Autodesk Fusion 360 part; units mm, degrees
(part 2 of 3)
  spline S36 degree 3 poles (-24.395426, -8.554265) (-24.395465, -8.554267) (-24.395536, -8.554312) (-24.395687, -8.554358) (-24.395947, -8.55446) (-24.39632, -8.554595) (-24.396767, -8.554761) (-24.397364, -8.55498) (-24.39811, -8.555255) (-24.399304, -8.555692) (-24.400799, -8.556237) (-24.402594, -8.556887) (-24.404391, -8.557534) (-24.406791, -8.558391) (-24.409796, -8.559455) (-24.413409, -8.560717) (-24.41824, -8.562383) (-24.4243, -8.56443) (-24.431601, -8.56683) (-24.438936, -8.569176) (-24.446305, -8.571466) (-24.456185, -8.574449) (-24.468619, -8.57804) (-24.483659, -8.582123) (-24.498834, -8.585986) (-24.519301, -8.590855) (-24.545236, -8.596386) (-24.576818, -8.602122) (-24.608947, -8.606975) (-24.641626, -8.610943) (-24.674857, -8.614028) (-24.708644, -8.616229) (-24.742988, -8.617551) (-24.780469, -8.617998) (-24.820659, -8.617471) (-24.876835, -8.6153) (-24.945324, -8.609872) (-25.025264, -8.598882) (-25.126818, -8.578556) (-25.247544, -8.542158) (-25.382434, -8.479922) (-25.505634, -8.399601) (-25.615962, -8.302262) (-25.71213, -8.190517) (-25.791503, -8.065677) (-25.85304, -7.928997) (-25.889046, -7.806726) (-25.914553, -7.676396) (-25.925922, -7.56615) (-25.929419, -7.42171) (-25.922149, -7.275178) (-25.893888, -7.104928) (-25.846241, -6.946475) (-25.779164, -6.799948) (-25.692713, -6.66553) (-25.623034, -6.584982) (-25.585516, -6.547045) knots 0 0 0 0 0.00001191 0.00002383 0.00004767 0.00009534 0.00014302 0.0001907 0.00028608 0.00038148 0.00057233 0.00076326 0.00095427 0.00114536 0.00152777 0.00191052 0.00229359 0.00306076 0.00382935 0.0045994 0.00537098 0.00614415 0.00769542 0.00925368 0.01081934 0.01239283 0.0155649 0.01877326 0.02202112 0.02531156 0.02864758 0.03203205 0.03546776 0.03895735 0.04327594 0.04752418 0.05582128 0.06387588 0.07171686 0.08687652 0.10158251 0.11613429 0.1308396 0.14557655 0.16021882 0.1750644 0.19040025 0.19833873 0.21488991 0.22356159 0.24167717 0.25880927 0.27521126 0.29116989 0.30699465 0.32300139 0.32300139 0.32300139 0.32300139
  spline S37 degree 3 poles (-25.585516, -6.547045) (-25.585469, -6.547019) (-25.585408, -6.546928) (-25.585253, -6.546786) (-25.584996, -6.54652) (-25.584621, -6.546149) (-25.584174, -6.5457) (-25.583577, -6.545104) (-25.582831, -6.544358) (-25.581635, -6.543167) (-25.580139, -6.541682) (-25.578341, -6.539903) (-25.57654, -6.53813) (-25.574135, -6.535772) (-25.571121, -6.532836) (-25.567491, -6.52933) (-25.562638, -6.524683) (-25.556542, -6.518921) (-25.549177, -6.512077) (-25.541764, -6.505308) (-25.534303, -6.498614) (-25.524299, -6.489793) (-25.511674, -6.478952) (-25.496325, -6.466233) (-25.480786, -6.453812) (-25.459829, -6.437659) (-25.433146, -6.418203) (-25.400347, -6.396037) (-25.366789, -6.375065) (-25.332474, -6.35529) (-25.297401, -6.336712) (-25.249516, -6.313481) (-25.187633, -6.287409) (-25.110548, -6.261018) (-25.03045, -6.239439) (-24.947346, -6.222675) (-24.83089, -6.206504) (-24.706133, -6.200325) (-24.576428, -6.204015) (-24.443025, -6.216082) (-24.315291, -6.240535) (-24.195161, -6.27832) (-24.110628, -6.312512) (-24.030429, -6.352955) (-23.954569, -6.399645) (-23.88306, -6.452573) (-23.815908, -6.511728) (-23.753121, -6.577091) (-23.714614, -6.624254) (-23.696116, -6.648755) knots 0 0 0 0 0.00001583 0.00003166 0.00006332 0.00012664 0.00018996 0.00025326 0.00037985 0.00050641 0.00075944 0.00101235 0.00126515 0.00151783 0.00202285 0.00252743 0.00303157 0.00403858 0.00504395 0.00604777 0.0070501 0.00805102 0.01004891 0.01204207 0.0140311 0.01601662 0.01997946 0.02393569 0.02789033 0.03184836 0.03581479 0.03979457 0.04781256 0.055942 0.06421981 0.07268094 0.08135818 0.09947342 0.11006808 0.12026679 0.1396396 0.14892549 0.15801382 0.16696446 0.17583997 0.18470439 0.1936219 0.20265543 0.21186547 0.21186547 0.21186547 0.21186547
  spline S38 degree 3 poles (-23.696116, -6.648755) (-23.696094, -6.648812) (-23.695999, -6.648897) (-23.695864, -6.649097) (-23.695601, -6.649434) (-23.69524, -6.649922) (-23.694801, -6.650505) (-23.694217, -6.651284) (-23.693488, -6.652258) (-23.692324, -6.653819) (-23.690871, -6.655773) (-23.689132, -6.658124) (-23.687398, -6.66048) (-23.685091, -6.66363) (-23.682219, -6.667582) (-23.678791, -6.672345) (-23.674243, -6.678729) (-23.668604, -6.686766) (-23.661915, -6.696493) (-23.655299, -6.70631) (-23.648756, -6.716216) (-23.640117, -6.729563) (-23.629502, -6.746475) (-23.617076, -6.767096) (-23.604944, -6.788075) (-23.593105, -6.809412) (-23.58156, -6.831107) (-23.566499, -6.860625) (-23.548409, -6.898443) (-23.527958, -6.945082) (-23.508681, -6.993157) (-23.490577, -7.042666) (-23.467785, -7.111241) (-23.442299, -7.200695) (-23.416694, -7.312775) (-23.395774, -7.430597) (-23.379532, -7.55417) (-23.365899, -7.706632) (-23.360337, -7.841833) (-23.359213, -7.984241) (-23.361184, -8.106853) (-23.370881, -8.296844) (-23.39479, -8.520005) (-23.444159, -8.769481) (-23.513751, -8.99517) (-23.603678, -9.196984) (-23.679006, -9.318219) (-23.719856, -9.373935) knots 0 0 0 0 0.00001823 0.00003647 0.00007294 0.0001459 0.00021888 0.00029186 0.00043785 0.00058389 0.0008761 0.00116849 0.00146105 0.00175379 0.00233982 0.00292658 0.0035141 0.00469142 0.00587191 0.00705566 0.00824278 0.00943337 0.01182537 0.0142325 0.01665555 0.01909531 0.02155255 0.02402802 0.02903642 0.03412638 0.03930334 0.04457246 0.04993864 0.06097948 0.07246123 0.08441435 0.0968659 0.10983987 0.13032478 0.1374365 0.15256362 0.16710419 0.19450011 0.2198151 0.24328444 0.26520232 0.28592841 0.28592841 0.28592841 0.28592841
  spline S39 degree 3 poles (-23.719856, -9.373935) (-23.71991, -9.373973) (-23.719966, -9.374101) (-23.720133, -9.374303) (-23.720323, -9.374573) (-23.720559, -9.37489) (-23.720871, -9.375315) (-23.721262, -9.375845) (-23.721888, -9.376693) (-23.722671, -9.377752) (-23.723612, -9.379021) (-23.724554, -9.380288) (-23.725811, -9.381975) (-23.727385, -9.38408) (-23.729279, -9.3866) (-23.731808, -9.389949) (-23.734981, -9.39412) (-23.738807, -9.399099) (-23.742651, -9.404053) (-23.746512, -9.40898) (-23.75168, -9.415509) (-23.758182, -9.423604) (-23.766061, -9.43322) (-23.774009, -9.44273) (-23.784684, -9.45525) (-23.798203, -9.47064) (-23.814727, -9.488709) (-23.831528, -9.506354) (-23.848606, -9.523575) (-23.865963, -9.540371) (-23.889436, -9.562165) (-23.91949, -9.58837) (-23.956721, -9.618165) (-23.995063, -9.64626) (-24.034514, -9.672655) (-24.088658, -9.705619) (-24.159327, -9.742656) (-24.248423, -9.780173) (-24.341926, -9.810837) (-24.439815, -9.834646) (-24.542078, -9.851609) (-24.648701, -9.861723) (-24.747073, -9.864653) (-24.834821, -9.862789) (-24.933295, -9.856099) (-25.05069, -9.839495) (-25.183656, -9.805449) (-25.306551, -9.757525) (-25.419202, -9.695724) (-25.487374, -9.64528) (-25.519396, -9.618055) knots 0 0 0 0 0.00001977 0.00003954 0.00007909 0.00011863 0.00015817 0.00023723 0.00031628 0.00047431 0.00063228 0.00079019 0.00094802 0.00126349 0.00157868 0.00189361 0.00252267 0.00315068 0.00377766 0.00440362 0.00502857 0.0062755 0.00751858 0.00875793 0.00999366 0.0124547 0.0149027 0.01733864 0.0197635 0.02217829 0.02458403 0.02937218 0.03413656 0.03888562 0.04362791 0.04837199 0.05789763 0.06753231 0.07734137 0.08738674 0.09772607 0.10841225 0.11949318 0.12723138 0.13473397 0.14909514 0.16273188 0.17582076 0.18856152 0.2011708 0.2011708 0.2011708 0.2011708
  spline S40 degree 3 poles (-25.519396, -9.618055) (-25.519451, -9.617994) (-25.519588, -9.617899) (-25.519834, -9.61768) (-25.520277, -9.617311) (-25.520903, -9.616775) (-25.521657, -9.616136) (-25.522659, -9.615281) (-25.52391, -9.614211) (-25.525906, -9.612496) (-25.528392, -9.610347) (-25.531362, -9.607758) (-25.534318, -9.60516) (-25.538238, -9.601684) (-25.543103, -9.597317) (-25.548887, -9.592035) (-25.556515, -9.58495) (-25.56591, -9.575999) (-25.576968, -9.565097) (-25.587798, -9.554045) (-25.5984, -9.542842) (-25.612215, -9.527724) (-25.628925, -9.508441) (-25.648089, -9.48467) (-25.666341, -9.460294) (-25.689459, -9.426989) (-25.716129, -9.383752) (-25.744449, -9.329455) (-25.769093, -9.272733) (-25.790057, -9.213591) (-25.80734, -9.152026) (-25.825721, -9.065562) (-25.833537, -8.998735) (-25.836416, -8.953505) knots 0 0 0 0 0.00002472 0.00004945 0.00009889 0.00019776 0.0002966 0.00039541 0.00059294 0.00079035 0.00118482 0.00157884 0.0019724 0.00236552 0.00315045 0.00393368 0.00471528 0.00627376 0.00782635 0.00937352 0.01091573 0.01245345 0.01551718 0.01856867 0.02161179 0.02465048 0.03072931 0.03683771 0.04300686 0.04926712 0.05564764 0.06217603 0.07577238 0.07577238 0.07577238 0.07577238
  line L18 (-25.836416, -8.953505) -> (-25.114226, -8.953505)
  spline S41 degree 3 poles (-25.114226, -8.953505) (-25.11419, -8.953651) (-25.114169, -8.953953) (-25.114074, -8.954546) (-25.113932, -8.955588) (-25.113713, -8.957071) (-25.113451, -8.958847) (-25.113093, -8.961207) (-25.112635, -8.964146) (-25.111878, -8.96882) (-25.110885, -8.974616) (-25.109616, -8.981513) (-25.108273, -8.988337) (-25.106389, -8.997303) (-25.103849, -9.00833) (-25.10049, -9.021325) (-25.095649, -9.038136) (-25.088861, -9.058451) (-25.079463, -9.081834) (-25.068871, -9.104039) (-25.057089, -9.125062) (-25.039898, -9.151358) (-25.015293, -9.18153) (-24.992387, -9.202475) (-24.980296, -9.212035) knots 0 0 0 0 0.00004513 0.00009023 0.00018037 0.00036035 0.00053995 0.00071917 0.00107647 0.00143227 0.00213939 0.00284064 0.00353611 0.00422592 0.00558893 0.00693059 0.00825183 0.01083675 0.01335229 0.01580753 0.01821221 0.0205767 0.02522625 0.02985048 0.02985048 0.02985048 0.02985048
  spline S42 degree 3 poles (-24.980296, -9.212035) (-24.98024, -9.212059) (-24.980157, -9.212156) (-24.979961, -9.212298) (-24.979632, -9.21257) (-24.979154, -9.212946) (-24.978582, -9.213401) (-24.977817, -9.214004) (-24.976858, -9.214756) (-24.975317, -9.215952) (-24.973379, -9.217436) (-24.971035, -9.219196) (-24.968672, -9.220937) (-24.965495, -9.223234) (-24.961476, -9.226058) (-24.956581, -9.229367) (-24.951611, -9.232598) (-24.946566, -9.235753) (-24.939725, -9.239866) (-24.93098, -9.244815) (-24.92021, -9.250433) (-24.909139, -9.255744) (-24.893881, -9.262459) (-24.874019, -9.270081) (-24.849141, -9.27794) (-24.823066, -9.284576) (-24.795795, -9.289992) (-24.767328, -9.294194) (-24.737664, -9.297183) (-24.712184, -9.298658) (-24.691216, -9.299244) (-24.673188, -9.299426) (-24.653232, -9.299089) (-24.624629, -9.297496) (-24.589832, -9.293544) (-24.549412, -9.285511) (-24.498098, -9.270573) (-24.437301, -9.243486) (-24.382506, -9.205403) (-24.337366, -9.16417) (-24.299649, -9.121493) (-24.274922, -9.08591) (-24.263196, -9.067085) knots 0 0 0 0 0.00001825 0.00003651 0.00007302 0.00014607 0.00021913 0.0002922 0.00043841 0.00058469 0.00087748 0.00117059 0.00146406 0.00175791 0.00234683 0.00293756 0.00353028 0.00412518 0.00472246 0.00592484 0.00713892 0.00836609 0.00960773 0.01213929 0.01474381 0.01743031 0.02020701 0.02308128 0.02605975 0.02914835 0.03073569 0.03235249 0.03455679 0.03672168 0.04094521 0.0450511 0.04906908 0.05696136 0.06489709 0.06896847 0.07528488 0.0819384 0.0819384 0.0819384 0.0819384
  spline S43 degree 3 poles (-24.263196, -9.067085) (-24.263147, -9.066977) (-24.263002, -9.066785) (-24.262763, -9.066376) (-24.262321, -9.06567) (-24.261702, -9.064654) (-24.260957, -9.063435) (-24.259967, -9.061803) (-24.258733, -9.059756) (-24.256768, -9.05646) (-24.254327, -9.05231) (-24.251431, -9.047284) (-24.248561, -9.042208) (-24.244762, -9.035354) (-24.240083, -9.026658) (-24.234592, -9.016047) (-24.229212, -9.005233) (-24.223942, -8.994216) (-24.217023, -8.979172) (-24.208654, -8.959849) (-24.199107, -8.935979) (-24.19, -8.911297) (-24.178306, -8.876904) (-24.164829, -8.831825) (-24.150594, -8.775109) (-24.138109, -8.715153) (-24.127368, -8.651956) (-24.118369, -8.585516) (-24.108476, -8.49056) (-24.104034, -8.417528) (-24.102136, -8.367785) knots 0 0 0 0 0.00003561 0.00007124 0.00014252 0.00028522 0.0004281 0.00057117 0.00085784 0.00114525 0.00172229 0.00230233 0.00288541 0.00347157 0.0046533 0.00584785 0.00705551 0.0082766 0.0095114 0.01202317 0.014593 0.01722287 0.01991463 0.02549015 0.03133236 0.03745197 0.04385828 0.05055936 0.05756225 0.07249603 0.07249603 0.07249603 0.07249603
  ellipse E2 centre (1150.427202, 948.865831) end of major axis (-13.478159, -21.350553) minor radius 28.956501 (-13.625826, -20.873205) -> (-13.473246, -21.356365) ccw
  spline S44 degree 3 poles (-13.473246, -21.356365) (-13.473203, -21.356392) (-13.473151, -21.356485) (-13.473011, -21.35663) (-13.472784, -21.356904) (-13.47245, -21.357284) (-13.472052, -21.357743) (-13.471521, -21.358354) (-13.470855, -21.359116) (-13.469789, -21.360332) (-13.468453, -21.361845) (-13.466843, -21.363653) (-13.465227, -21.365451) (-13.463065, -21.367834) (-13.460349, -21.37079) (-13.457063, -21.3743) (-13.452656, -21.378925) (-13.447086, -21.384612) (-13.4403, -21.391291) (-13.433419, -21.397818) (-13.426443, -21.404192) (-13.417028, -21.412475) (-13.405014, -21.422455) (-13.390196, -21.433835) (-13.374995, -21.444604) (-13.354214, -21.458147) (-13.32721, -21.473579) (-13.293279, -21.489621) (-13.257808, -21.503193) (-13.220801, -21.514291) (-13.182256, -21.522914) (-13.142173, -21.529062) (-13.100551, -21.532728) (-13.058754, -21.533904) (-13.017801, -21.532771) (-12.966494, -21.52815) (-12.90562, -21.516609) (-12.837479, -21.492778) (-12.775443, -21.459112) (-12.719626, -21.415643) (-12.687275, -21.380934) (-12.672226, -21.362295) knots 0 0 0 0 0.0000152 0.0000304 0.00006079 0.00012156 0.00018231 0.00024304 0.00036444 0.00048576 0.00072815 0.00097023 0.00121199 0.00145344 0.00193543 0.00241625 0.00289592 0.003852 0.004804 0.00575224 0.00669705 0.00763876 0.00951415 0.01138119 0.01324267 0.01510137 0.01882097 0.02256319 0.02635022 0.03020356 0.03414371 0.03818995 0.04236016 0.04667078 0.05072716 0.05464318 0.06211749 0.06924962 0.07621391 0.083197 0.09038387 0.09038387 0.09038387 0.09038387
  spline S45 degree 3 poles (-12.672226, -21.362295) (-12.672221, -21.362272) (-12.672176, -21.362241) (-12.672124, -21.362163) (-12.672015, -21.362035) (-12.671869, -21.361847) (-12.67169, -21.361624) (-12.671452, -21.361325) (-12.671155, -21.360952) (-12.67068, -21.360354) (-12.670088, -21.359605) (-12.669379, -21.358705) (-12.668672, -21.357802) (-12.667732, -21.356597) (-12.666562, -21.355085) (-12.665165, -21.353264) (-12.663312, -21.350826) (-12.661014, -21.34776) (-12.658287, -21.344052) (-12.65559, -21.340315) (-12.652922, -21.336549) (-12.649403, -21.331484) (-12.645078, -21.325078) (-12.640011, -21.317281) (-12.635064, -21.309366) (-12.628612, -21.298633) (-12.620844, -21.284916) (-12.612021, -21.268021) (-12.603675, -21.250656) (-12.595807, -21.232821) (-12.588417, -21.214516) (-12.579133, -21.189299) (-12.568738, -21.156541) (-12.558269, -21.115632) (-12.549712, -21.072837) (-12.543068, -21.028153) (-12.538331, -20.981578) (-12.535514, -20.933107) (-12.53459, -20.884412) (-12.535534, -20.836698) (-12.539453, -20.777064) (-12.549124, -20.706563) (-12.569038, -20.627415) (-12.592673, -20.566619) (-12.618371, -20.516533) (-12.644379, -20.475234) (-12.681753, -20.42818) (-12.728762, -20.382664) (-12.787141, -20.341886) (-12.852106, -20.310359) (-12.923533, -20.288054) (-13.001358, -20.274891) (-13.09578, -20.270209) (-13.176999, -20.276108) (-13.252832, -20.291712) (-13.310791, -20.309785) (-13.375015, -20.340819) (-13.432929, -20.380944) (-13.466838, -20.413326) (-13.482576, -20.430735) knots 0 0 0 0 0.00000715 0.00001431 0.00002862 0.00005725 0.00008587 0.0001145 0.00017176 0.00022903 0.00034359 0.00045817 0.00057278 0.00068743 0.0009168 0.0011463 0.00137593 0.0018356 0.00229584 0.00275669 0.00321819 0.00368038 0.00460695 0.00553671 0.00646995 0.00740696 0.00929337 0.01119826 0.0131238 0.01507212 0.01704527 0.01904521 0.02313256 0.0273489 0.03170726 0.03621948 0.04089625 0.04574722 0.05078106 0.05550411 0.06005954 0.06870514 0.0768121 0.08449091 0.08821165 0.09368971 0.09910183 0.10620576 0.11323827 0.12037497 0.12778318 0.13561204 0.14398747 0.15610626 0.15990029 0.16720338 0.17425492 0.18121652 0.18825692 0.18825692 0.18825692 0.18825692
  spline S46 degree 3 poles (-13.482576, -20.430735) (-13.482627, -20.430812) (-13.482768, -20.430938) (-13.483009, -20.43122) (-13.48345, -20.4317) (-13.484068, -20.432394) (-13.484812, -20.433226) (-13.4858, -20.434337) (-13.487031, -20.435731) (-13.48899, -20.43797) (-13.491419, -20.440786) (-13.494302, -20.444192) (-13.497154, -20.447625) (-13.500915, -20.452239) (-13.505538, -20.458075) (-13.51096, -20.465186) (-13.518027, -20.474819) (-13.52655, -20.487138) (-13.536267, -20.502341) (-13.545481, -20.517976) (-13.554194, -20.534045) (-13.565195, -20.556152) (-13.577695, -20.584933) (-13.59061, -20.621025) (-13.601521, -20.658844) (-13.613595, -20.712434) (-13.623467, -20.784087) (-13.625826, -20.842827) (-13.625826, -20.873205) knots 0 0 0 0 0.0000279 0.00005579 0.00011158 0.00022316 0.00033474 0.00044631 0.00066944 0.00089255 0.00133877 0.001785 0.00223128 0.00267766 0.00357082 0.00446482 0.00535996 0.0071548 0.00895787 0.01077156 0.01259824 0.01444021 0.0181784 0.02200385 0.02593251 0.02997909 0.03847552 0.04758904 0.04758904 0.04758904 0.04758904
  ellipse E3 centre (-5.783059, -31.50099) end of major axis (1.947224, -43.157824) minor radius 3.336725 (-13.346096, -19.759405) -> (-13.638536, -19.946735) ccw
  spline S47 degree 3 poles (-13.346096, -19.759405) (-13.345943, -19.759371) (-13.345658, -19.759234) (-13.345066, -19.759032) (-13.344334, -19.758756) (-13.343451, -19.758436) (-13.342274, -19.758006) (-13.340801, -19.757473) (-13.338442, -19.756623) (-13.335487, -19.75557) (-13.331933, -19.75432) (-13.328371, -19.753084) (-13.323606, -19.751453) (-13.317628, -19.749449) (-13.310423, -19.747101) (-13.300757, -19.74404) (-13.288584, -19.740351) (-13.27385, -19.736148) (-13.258974, -19.732165) (-13.243954, -19.7284) (-13.223675, -19.723657) (-13.197953, -19.718276) (-13.1666, -19.712708) (-13.134665, -19.708006) (-13.090973, -19.702849) (-13.046404, -19.699479) (-13.001045, -19.697797) (-12.963551, -19.697366) (-12.923291, -19.697885) (-12.866956, -19.700041) (-12.798256, -19.705425) (-12.718051, -19.716326) (-12.616146, -19.736485) (-12.495018, -19.772563) (-12.359664, -19.834267) (-12.236137, -19.913885) (-12.162529, -19.978213) (-12.128036, -20.012845) knots 0 0 0 0 0.00004693 0.00009387 0.00018776 0.00028168 0.00037561 0.00056355 0.00075159 0.00112793 0.00150464 0.00188174 0.00225922 0.00301539 0.0037732 0.00453272 0.00605709 0.00758897 0.00912881 0.01067706 0.01223416 0.01537652 0.01855933 0.02178578 0.02505896 0.03175648 0.03518688 0.03867491 0.04300442 0.04726431 0.05558625 0.06366654 0.0715326 0.08673495 0.10146408 0.11600988 0.13067364 0.13067364 0.13067364 0.13067364
  spline S48 degree 3 poles (-12.128036, -20.012845) (-12.128013, -20.012887) (-12.127928, -20.012944) (-12.127799, -20.013087) (-12.127555, -20.013323) (-12.127216, -20.013667) (-12.126805, -20.014077) (-12.126259, -20.014626) (-12.125577, -20.015312) (-12.124487, -20.01641) (-12.123128, -20.017784) (-12.1215, -20.019437) (-12.119877, -20.021092) (-12.11772, -20.023303) (-12.115033, -20.026073) (-12.111825, -20.02941) (-12.107573, -20.033873) (-12.1023, -20.039481) (-12.096038, -20.046259) (-12.089845, -20.053084) (-12.083721, -20.059954) (-12.07565, -20.069173) (-12.065731, -20.080812) (-12.054097, -20.094973) (-12.042735, -20.109319) (-12.027958, -20.128686) (-12.010161, -20.153373) (-11.989893, -20.183749) (-11.970721, -20.214867) (-11.952646, -20.246728) (-11.935667, -20.279332) (-11.914425, -20.32393) (-11.890596, -20.38166) (-11.866501, -20.453674) (-11.846806, -20.528648) (-11.831512, -20.60658) (-11.816751, -20.716092) (-11.811266, -20.830901) (-11.814237, -20.948177) (-11.82355, -21.065374) (-11.846795, -21.205355) (-11.894436, -21.363801) (-11.961513, -21.510332) (-12.047965, -21.64475) (-12.117646, -21.725298) (-12.155166, -21.763235) knots 0 0 0 0 0.00001451 0.00002903 0.00005806 0.00011611 0.00017416 0.0002322 0.00034827 0.00046431 0.00069633 0.00092825 0.00116008 0.00139182 0.00185502 0.00231787 0.00278037 0.00370437 0.0046271 0.00554863 0.00646902 0.00738836 0.00922414 0.01105658 0.01288626 0.01471378 0.01836458 0.02201391 0.02566655 0.02932729 0.03300088 0.036692 0.04414416 0.05172095 0.05945658 0.06738327 0.07553092 0.09259101 0.10178952 0.11071367 0.12784603 0.14424814 0.16020682 0.17603166 0.19203863 0.19203863 0.19203863 0.19203863
  spline S49 degree 3 poles (-12.155166, -21.763235) (-12.155212, -21.763261) (-12.155273, -21.763352) (-12.155428, -21.763494) (-12.155684, -21.76376) (-12.156057, -21.764131) (-12.156502, -21.76458) (-12.157097, -21.765176) (-12.157841, -21.765922) (-12.159032, -21.767113) (-12.160522, -21.768598) (-12.162314, -21.770377) (-12.164109, -21.77215) (-12.166505, -21.774508) (-12.169509, -21.777444) (-12.173125, -21.78095) (-12.177962, -21.785597) (-12.184037, -21.79136) (-12.191378, -21.798203) (-12.198768, -21.804972) (-12.206205, -21.811666) (-12.216179, -21.820487) (-12.228768, -21.831328) (-12.244076, -21.844048) (-12.259575, -21.856469) (-12.280482, -21.872621) (-12.307107, -21.892078) (-12.339842, -21.914245) (-12.373343, -21.935216) (-12.407607, -21.954991) (-12.442635, -21.973569) (-12.490471, -21.996802) (-12.552303, -22.022874) (-12.629343, -22.049264) (-12.70941, -22.070842) (-12.792492, -22.087607) (-12.87858, -22.099557) (-12.967668, -22.106701) (-13.063476, -22.109104) (-13.163638, -22.106265) (-13.297394, -22.094185) (-13.425517, -22.069697) (-13.546052, -22.031836) (-13.630903, -21.997554) (-13.71142, -21.956985) (-13.787592, -21.910128) (-13.859403, -21.856984) (-13.926839, -21.797559) (-13.989887, -21.731867) (-14.02854, -21.684452) (-14.047106, -21.659815) knots 0 0 0 0 0.0000158 0.0000316 0.00006321 0.00012641 0.0001896 0.00025279 0.00037915 0.00050547 0.00075804 0.00101049 0.00126282 0.00151504 0.00201915 0.00252282 0.00302605 0.00403127 0.00503488 0.00603695 0.00703756 0.00803678 0.01003136 0.0120213 0.01400722 0.01598974 0.01994687 0.02389784 0.02784764 0.03180128 0.03576374 0.03973997 0.04775209 0.05587719 0.06415198 0.07261123 0.08128746 0.09021082 0.099409 0.1100268 0.12025147 0.13968263 0.14900009 0.15812123 0.16710586 0.17601663 0.18491787 0.19387418 0.20294913 0.21220391 0.21220391 0.21220391 0.21220391
  spline S50 degree 3 poles (-14.047106, -21.659815) (-14.047128, -21.659758) (-14.047223, -21.659673) (-14.04736, -21.659473) (-14.047624, -21.659136) (-14.047988, -21.658648) (-14.048431, -21.658065) (-14.049018, -21.657286) (-14.049753, -21.656312) (-14.050926, -21.654752) (-14.05239, -21.652797) (-14.054142, -21.650447) (-14.05589, -21.64809) (-14.058214, -21.64494) (-14.061108, -21.640989) (-14.064561, -21.636226) (-14.067996, -21.631441) (-14.071412, -21.626634) (-14.075945, -21.62019) (-14.081565, -21.612079) (-14.088231, -21.602263) (-14.094823, -21.592357) (-14.103527, -21.579011) (-14.114222, -21.562101) (-14.126742, -21.541482) (-14.138966, -21.520505) (-14.150894, -21.499171) (-14.162527, -21.477479) (-14.177701, -21.447969) (-14.195926, -21.410164) (-14.216532, -21.36354) (-14.235955, -21.315487) (-14.254196, -21.266004) (-14.277156, -21.197483) (-14.302833, -21.108114) (-14.328633, -20.99616) (-14.349711, -20.878504) (-14.366076, -20.755146) (-14.379812, -20.603015) (-14.385419, -20.46814) (-14.38655, -20.3261) (-14.384576, -20.203794) (-14.37487, -20.014196) (-14.350914, -19.791389) (-14.3014, -19.542203) (-14.231519, -19.316654) (-14.141106, -19.11488) (-14.065326, -18.993714) (-14.024216, -18.938035) knots 0 0 0 0 0.00001828 0.00003657 0.00007314 0.0001463 0.00021947 0.00029265 0.00043904 0.00058547 0.00087847 0.00117163 0.00146497 0.00175848 0.00234603 0.0029343 0.0035233 0.00411304 0.00470355 0.00588688 0.0070734 0.00826321 0.00945642 0.01185344 0.01426527 0.01669273 0.01913659 0.02159763 0.02407659 0.02909102 0.03418575 0.03936621 0.04463752 0.05000459 0.06104314 0.07251706 0.0844566 0.09688856 0.10983668 0.13027045 0.13736168 0.15244997 0.16695826 0.19430734 0.2195969 0.24306072 0.26499326 0.28575655 0.28575655 0.28575655 0.28575655
  spline S51 degree 3 poles (-14.024216, -18.938035) (-14.024189, -18.938016) (-14.02416, -18.937951) (-14.024076, -18.93785) (-14.023942, -18.93766) (-14.023743, -18.937395) (-14.023508, -18.937074) (-14.023193, -18.936648) (-14.022799, -18.936115) (-14.022169, -18.935263) (-14.02138, -18.934198) (-14.020433, -18.932923) (-14.019484, -18.931649) (-14.018218, -18.929953) (-14.016633, -18.927837) (-14.014727, -18.925305) (-14.01218, -18.921938) (-14.008985, -18.917746) (-14.005133, -18.912741) (-14.001263, -18.907763) (-13.997376, -18.902811) (-13.992175, -18.89625) (-13.985631, -18.888114) (-13.977702, -18.878451) (-13.969704, -18.868895) (-13.958963, -18.856315) (-13.945364, -18.840853) (-13.928745, -18.822701) (-13.91185, -18.804977) (-13.89468, -18.78768) (-13.877233, -18.770812) (-13.853642, -18.748929) (-13.823445, -18.72262) (-13.786043, -18.692712) (-13.747534, -18.664516) (-13.707919, -18.638034) (-13.653563, -18.604968) (-13.582629, -18.567829) (-13.493211, -18.530222) (-13.39938, -18.499499) (-13.301151, -18.475655) (-13.198532, -18.458675) (-13.091528, -18.448557) (-12.993035, -18.445631) (-12.905433, -18.447479) (-12.807516, -18.454103) (-12.690802, -18.470551) (-12.558603, -18.504315) (-12.436406, -18.551889) (-12.324357, -18.613299) (-12.256535, -18.66345) (-12.224666, -18.690525) knots 0 0 0 0 0.00000994 0.00001988 0.00003978 0.00007955 0.00011933 0.0001591 0.00023862 0.00031813 0.00047709 0.00063598 0.00079481 0.00095356 0.00127086 0.00158788 0.00190463 0.0025373 0.0031689 0.00379944 0.00442893 0.00505739 0.00631127 0.00756118 0.00880726 0.01004961 0.01252362 0.01498419 0.01743233 0.01986904 0.02229533 0.02471223 0.02952182 0.0343065 0.03907489 0.04383565 0.04859751 0.05815709 0.06782455 0.07766628 0.08774516 0.09811974 0.10884363 0.11996535 0.1276613 0.13512168 0.1493991 0.16295401 0.17596474 0.18863321 0.20117846 0.20117846 0.20117846 0.20117846
  spline S52 degree 3 poles (-12.224666, -18.690525) (-12.224611, -18.690586) (-12.224474, -18.69068) (-12.224229, -18.690898) (-12.223788, -18.691265) (-12.223165, -18.691798) (-12.222415, -18.692435) (-12.221417, -18.693285) (-12.220172, -18.694349) (-12.218185, -18.696056) (-12.21571, -18.698194) (-12.212754, -18.700771) (-12.209812, -18.703357) (-12.205911, -18.706817) (-12.20107, -18.711166) (-12.195315, -18.716426) (-12.187725, -18.723483) (-12.17838, -18.732403) (-12.167384, -18.743272) (-12.156617, -18.754295) (-12.146079, -18.765472) (-12.132349, -18.780564) (-12.115747, -18.799825) (-12.096715, -18.823582) (-12.078596, -18.847959) (-12.055646, -18.881297) (-12.029181, -18.924615) (-12.001093, -18.979048) (-11.976646, -19.035956) (-11.955833, -19.095332) (-11.93864, -19.157178) (-11.920279, -19.244108) (-11.91236, -19.311288) (-11.909346, -19.356775) knots 0 0 0 0 0.0000246 0.00004921 0.00009842 0.00019682 0.00029519 0.00039353 0.00059012 0.00078659 0.0011792 0.00157136 0.00196308 0.00235436 0.00313564 0.00391527 0.0046933 0.00624481 0.00779065 0.00933132 0.0108673 0.01239908 0.01545192 0.01849396 0.02152923 0.02456179 0.03063395 0.0367436 0.04292214 0.04919979 0.05560524 0.06216532 0.07584137 0.07584137 0.07584137 0.07584137
  line L19 (-11.909346, -19.356775) -> (-12.626456, -19.354225)
  spline S53 degree 3 poles (-12.626456, -19.354225) (-12.626492, -19.35408) (-12.626516, -19.35378) (-12.626614, -19.353191) (-12.626764, -19.352158) (-12.626994, -19.350686) (-12.627269, -19.348923) (-12.627642, -19.346581) (-12.62812, -19.343666) (-12.628907, -19.339031) (-12.629935, -19.333284) (-12.631242, -19.326447) (-12.63262, -19.319685) (-12.634544, -19.310807) (-12.637125, -19.299894) (-12.640521, -19.287041) (-12.645394, -19.270433) (-12.652192, -19.250387) (-12.661574, -19.227343) (-12.672122, -19.205496) (-12.683844, -19.184848) (-12.700945, -19.159068) (-12.725462, -19.129551) (-12.74831, -19.109195) (-12.760376, -19.099935) knots 0 0 0 0 0.00004484 0.00008967 0.00017923 0.00035807 0.00053651 0.00071456 0.00106948 0.00142284 0.00212493 0.00282093 0.00351095 0.00419508 0.00554613 0.006875 0.00818265 0.01073811 0.01322147 0.01564229 0.01801099 0.02033878 0.02491669 0.0294796 0.0294796 0.0294796 0.0294796
  spline S54 degree 3 poles (-12.760376, -19.099935) (-12.760431, -19.099913) (-12.760514, -19.099819) (-12.76071, -19.099684) (-12.761039, -19.099423) (-12.761518, -19.099064) (-12.762089, -19.098629) (-12.762855, -19.098051) (-12.763814, -19.097332) (-12.765356, -19.096188) (-12.767296, -19.094768) (-12.769642, -19.093084) (-12.772007, -19.091417) (-12.775189, -19.089218) (-12.779216, -19.086514) (-12.784121, -19.083345) (-12.79078, -19.079207) (-12.799302, -19.074215) (-12.809812, -19.068532) (-12.820631, -19.063141) (-12.831759, -19.058042) (-12.847119, -19.051585) (-12.867128, -19.044252) (-12.892198, -19.036687) (-12.918501, -19.03029) (-12.946034, -19.025063) (-12.9748, -19.021002) (-13.004797, -19.01811) (-13.030575, -19.016681) (-13.051802, -19.016113) (-13.069997, -19.015934) (-13.09008, -19.016273) (-13.118778, -19.017882) (-13.153651, -19.02187) (-13.194108, -19.029972) (-13.245345, -19.045014) (-13.30589, -19.072256) (-13.360256, -19.110536) (-13.404826, -19.151912) (-13.441898, -19.194675) (-13.466064, -19.230295) (-13.477486, -19.249125) knots 0 0 0 0 0.00001795 0.0000359 0.0000718 0.00014363 0.00021549 0.00028737 0.00043122 0.00057519 0.00086348 0.00115226 0.00144157 0.00173142 0.00231282 0.00289668 0.00348316 0.00466468 0.00585883 0.00706699 0.00829044 0.00953048 0.0120648 0.01467936 0.01738248 0.02018166 0.02308367 0.02609459 0.02921985 0.03082698 0.03246447 0.03467839 0.03685122 0.0410857 0.04519638 0.04921342 0.05708839 0.06498957 0.06903834 0.07531483 0.08192171 0.08192171 0.08192171 0.08192171
  spline S55 degree 3 poles (-13.477486, -19.249125) (-13.477534, -19.249233) (-13.477675, -19.249427) (-13.477911, -19.249838) (-13.478345, -19.250547) (-13.478952, -19.251569) (-13.479684, -19.252794) (-13.480657, -19.254435) (-13.481869, -19.256493) (-13.483801, -19.259804) (-13.486199, -19.263975) (-13.489047, -19.269022) (-13.491868, -19.27412) (-13.495604, -19.281001) (-13.500208, -19.289729) (-13.505612, -19.300373) (-13.512716, -19.31491) (-13.521327, -19.333589) (-13.531181, -19.356676) (-13.540613, -19.38056) (-13.549623, -19.405239) (-13.561208, -19.439607) (-13.574595, -19.484614) (-13.588796, -19.541195) (-13.601318, -19.600965) (-13.612166, -19.663927) (-13.621343, -19.730085) (-13.631572, -19.824578) (-13.636367, -19.897244) (-13.638536, -19.946735) knots 0 0 0 0 0.00003558 0.00007117 0.00014239 0.00028496 0.00042771 0.00057065 0.00085707 0.00114422 0.00172076 0.00230031 0.00288291 0.00346859 0.00464936 0.00584293 0.00704959 0.00950322 0.01201248 0.01457938 0.01720578 0.01989345 0.02545867 0.03128727 0.03738958 0.04377463 0.05045029 0.05742351 0.07228503 0.07228503 0.07228503 0.07228503
  line L20 (-30.972226, -31.397235) -> (-31.109706, -31.317855)
  spline S56 degree 3 poles (-31.109706, -31.317855) (-31.109736, -31.317824) (-31.109821, -31.317794) (-31.109965, -31.317701) (-31.11023, -31.317553) (-31.1106, -31.317333) (-31.111046, -31.317071) (-31.111637, -31.316717) (-31.112372, -31.316272) (-31.113539, -31.315551) (-31.114983, -31.314633) (-31.116693, -31.313506) (-31.118377, -31.312353) (-31.120587, -31.310785) (-31.123287, -31.308765) (-31.12643, -31.306243) (-31.130475, -31.302766) (-31.13528, -31.298199) (-31.140639, -31.292379) (-31.145571, -31.286258) (-31.150071, -31.27986) (-31.155476, -31.27101) (-31.161133, -31.259361) (-31.166086, -31.244664) (-31.169146, -31.229456) (-31.170635, -31.208723) (-31.167406, -31.182263) (-31.159234, -31.162399) (-31.153856, -31.153085) knots 0 0 0 0 0.00001296 0.00002591 0.00005181 0.00010357 0.00015528 0.00020695 0.00031013 0.00041314 0.0006186 0.00082337 0.00102747 0.00123094 0.00163605 0.00203893 0.00243978 0.00323597 0.0040261 0.00481132 0.00559265 0.00637096 0.00792065 0.00946615 0.01101166 0.01256136 0.01568806 0.01891458 0.01891458 0.01891458 0.01891458
  line L21 (-31.153856, -31.153085) -> (-30.024486, -29.196945)
  spline S57 degree 3 poles (-30.024486, -29.196945) (-30.024455, -29.196915) (-30.024425, -29.19683) (-30.024332, -29.196685) (-30.024184, -29.196421) (-30.023964, -29.196051) (-30.023701, -29.195605) (-30.023348, -29.195014) (-30.022902, -29.194279) (-30.022181, -29.193112) (-30.021263, -29.191668) (-30.020135, -29.189958) (-30.018982, -29.188273) (-30.017414, -29.186064) (-30.015393, -29.183364) (-30.01287, -29.180221) (-30.009393, -29.176175) (-30.004825, -29.17137) (-29.999005, -29.166012) (-29.992883, -29.161079) (-29.986484, -29.156579) (-29.977633, -29.151174) (-29.965983, -29.145518) (-29.951286, -29.140565) (-29.936078, -29.137505) (-29.915344, -29.136015) (-29.888884, -29.139244) (-29.869019, -29.147417) (-29.859706, -29.152795) knots 0 0 0 0 0.00001296 0.00002591 0.00005181 0.00010358 0.00015529 0.00020696 0.00031016 0.00041317 0.00061865 0.00082343 0.00102755 0.00123104 0.00163618 0.00203909 0.00243997 0.00323623 0.00402641 0.00481169 0.00559308 0.00637144 0.00792121 0.00946679 0.01101235 0.01256208 0.01568881 0.01891534 0.01891534 0.01891534 0.01891534
  line L22 (-29.859706, -29.152795) -> (-29.722226, -29.232165)
  spline S58 degree 3 poles (-29.722226, -29.232165) (-29.722195, -29.232196) (-29.72211, -29.232226) (-29.721966, -29.232319) (-29.721702, -29.232467) (-29.721331, -29.232687) (-29.720886, -29.23295) (-29.720295, -29.233303) (-29.71956, -29.233748) (-29.718392, -29.23447) (-29.716948, -29.235388) (-29.715239, -29.236516) (-29.713554, -29.237669) (-29.711345, -29.239237) (-29.708645, -29.241257) (-29.705501, -29.24378) (-29.701456, -29.247257) (-29.696651, -29.251825) (-29.691293, -29.257646) (-29.68636, -29.263768) (-29.68186, -29.270166) (-29.676455, -29.279017) (-29.670798, -29.290667) (-29.665845, -29.305365) (-29.662786, -29.320573) (-29.661296, -29.341307) (-29.664525, -29.367767) (-29.672697, -29.387631) (-29.678076, -29.396945) knots 0 0 0 0 0.00001296 0.00002591 0.00005181 0.00010358 0.00015529 0.00020696 0.00031016 0.00041317 0.00061865 0.00082343 0.00102755 0.00123104 0.00163618 0.00203909 0.00243997 0.00323623 0.00402641 0.00481169 0.00559308 0.00637144 0.00792121 0.00946679 0.01101235 0.01256208 0.01568881 0.01891534 0.01891534 0.01891534 0.01891534
  line L23 (-29.678076, -29.396945) -> (-30.807446, -31.353085)
  spline S59 degree 3 poles (-30.807446, -31.353085) (-30.807476, -31.353115) (-30.807506, -31.3532) (-30.807599, -31.353345) (-30.807747, -31.353609) (-30.807968, -31.353979) (-30.80823, -31.354425) (-30.808584, -31.355016) (-30.809029, -31.355751) (-30.809751, -31.356918) (-30.810668, -31.358362) (-30.811796, -31.360072) (-30.812949, -31.361757) (-30.814517, -31.363966) (-30.816538, -31.366666) (-30.819061, -31.369809) (-30.822538, -31.373854) (-30.827106, -31.378659) (-30.832926, -31.384017) (-30.839048, -31.388949) (-30.845447, -31.393449) (-30.854298, -31.398853) (-30.865948, -31.404509) (-30.880646, -31.409461) (-30.895854, -31.412521) (-30.916587, -31.41401) (-30.943047, -31.410782) (-30.962912, -31.402612) (-30.972226, -31.397235) knots 0 0 0 0 0.00001296 0.00002591 0.00005181 0.00010358 0.00015529 0.00020696 0.00031016 0.00041317 0.00061865 0.00082343 0.00102755 0.00123103 0.00163617 0.00203907 0.00243994 0.00323617 0.00402634 0.00481159 0.00559296 0.0063713 0.00792103 0.00946659 0.01101214 0.01256187 0.01568859 0.01891498 0.01891498 0.01891498 0.01891498
  line L24 (-19.427876, -11.401835) -> (-19.565356, -11.322455)
  spline S60 degree 3 poles (-19.565356, -11.322455) (-19.565386, -11.322424) (-19.565471, -11.322394) (-19.565615, -11.322301) (-19.56588, -11.322153) (-19.56625, -11.321933) (-19.566696, -11.321671) (-19.567287, -11.321317) (-19.568022, -11.320872) (-19.569189, -11.320151) (-19.570633, -11.319233) (-19.572343, -11.318106) (-19.574027, -11.316953) (-19.576237, -11.315385) (-19.578937, -11.313365) (-19.58208, -11.310843) (-19.586125, -11.307366) (-19.59093, -11.302799) (-19.596289, -11.296979) (-19.601221, -11.290858) (-19.605721, -11.28446) (-19.611126, -11.27561) (-19.616783, -11.263961) (-19.621736, -11.249264) (-19.624796, -11.234056) (-19.626285, -11.213323) (-19.623056, -11.186863) (-19.614884, -11.166999) (-19.609506, -11.157685) knots 0 0 0 0 0.00001296 0.00002591 0.00005181 0.00010357 0.00015528 0.00020695 0.00031013 0.00041314 0.0006186 0.00082337 0.00102747 0.00123094 0.00163605 0.00203893 0.00243978 0.00323597 0.0040261 0.00481132 0.00559265 0.00637096 0.00792065 0.00946615 0.01101166 0.01256136 0.01568806 0.01891458 0.01891458 0.01891458 0.01891458
  line L25 (-19.609506, -11.157685) -> (-18.480136, -9.201545)
  spline S61 degree 3 poles (-18.480136, -9.201545) (-18.480105, -9.201515) (-18.480075, -9.20143) (-18.479982, -9.201285) (-18.479834, -9.201021) (-18.479614, -9.200651) (-18.479351, -9.200205) (-18.478998, -9.199614) (-18.478552, -9.198879) (-18.477831, -9.197712) (-18.476913, -9.196268) (-18.475785, -9.194558) (-18.474632, -9.192873) (-18.473064, -9.190664) (-18.471043, -9.187964) (-18.46852, -9.184821) (-18.465043, -9.180775) (-18.460475, -9.17597) (-18.454655, -9.170612) (-18.448533, -9.165679) (-18.442134, -9.161179) (-18.433283, -9.155774) (-18.421633, -9.150118) (-18.406936, -9.145165) (-18.391728, -9.142105) (-18.370994, -9.140615) (-18.344534, -9.143844) (-18.324669, -9.152017) (-18.315356, -9.157395) knots 0 0 0 0 0.00001296 0.00002591 0.00005181 0.00010358 0.00015529 0.00020696 0.00031016 0.00041317 0.00061865 0.00082343 0.00102755 0.00123104 0.00163618 0.00203909 0.00243997 0.00323623 0.00402641 0.00481169 0.00559308 0.00637144 0.00792121 0.00946679 0.01101235 0.01256208 0.01568881 0.01891534 0.01891534 0.01891534 0.01891534
  line L26 (-18.315356, -9.157395) -> (-18.177876, -9.236765)
  spline S62 degree 3 poles (-18.177876, -9.236765) (-18.177845, -9.236796) (-18.17776, -9.236826) (-18.177616, -9.236919) (-18.177352, -9.237067) (-18.176981, -9.237287) (-18.176536, -9.23755) (-18.175945, -9.237903) (-18.17521, -9.238348) (-18.174042, -9.23907) (-18.172598, -9.239988) (-18.170889, -9.241116) (-18.169204, -9.242269) (-18.166995, -9.243837) (-18.164295, -9.245857) (-18.161151, -9.24838) (-18.157106, -9.251857) (-18.152301, -9.256425) (-18.146943, -9.262246) (-18.14201, -9.268368) (-18.13751, -9.274766) (-18.132105, -9.283617) (-18.126448, -9.295267) (-18.121495, -9.309965) (-18.118436, -9.325173) (-18.116946, -9.345907) (-18.120175, -9.372367) (-18.128347, -9.392231) (-18.133726, -9.401545) knots 0 0 0 0 0.00001296 0.00002591 0.00005181 0.00010358 0.00015529 0.00020696 0.00031016 0.00041317 0.00061865 0.00082343 0.00102755 0.00123104 0.00163618 0.00203909 0.00243997 0.00323623 0.00402641 0.00481169 0.00559308 0.00637144 0.00792121 0.00946679 0.01101235 0.01256208 0.01568881 0.01891534 0.01891534 0.01891534 0.01891534
  line L27 (-18.133726, -9.401545) -> (-19.263096, -11.357685)
  spline S63 degree 3 poles (-19.263096, -11.357685) (-19.263126, -11.357715) (-19.263156, -11.3578) (-19.263249, -11.357945) (-19.263397, -11.358209) (-19.263618, -11.358579) (-19.26388, -11.359025) (-19.264234, -11.359616) (-19.264679, -11.360351) (-19.265401, -11.361518) (-19.266318, -11.362962) (-19.267446, -11.364672) (-19.268599, -11.366357) (-19.270167, -11.368566) (-19.272188, -11.371266) (-19.274711, -11.374409) (-19.278188, -11.378454) (-19.282756, -11.383259) (-19.288576, -11.388617) (-19.294698, -11.393549) (-19.301097, -11.398049) (-19.309948, -11.403453) (-19.321598, -11.409109) (-19.336296, -11.414061) (-19.351504, -11.417121) (-19.372237, -11.41861) (-19.398697, -11.415382) (-19.418562, -11.407212) (-19.427876, -11.401835) knots 0 0 0 0 0.00001296 0.00002591 0.00005181 0.00010358 0.00015529 0.00020696 0.00031016 0.00041317 0.00061865 0.00082343 0.00102755 0.00123103 0.00163617 0.00203907 0.00243994 0.00323617 0.00402634 0.00481159 0.00559296 0.0063713 0.00792103 0.00946659 0.01101214 0.01256187 0.01568859 0.01891498 0.01891498 0.01891498 0.01891498
  line L28 (-35.684336, -26.743225) -> (-35.763716, -26.605745)
  spline S64 degree 3 poles (-35.763716, -26.605745) (-35.763711, -26.605742) (-35.763739, -26.60572) (-35.763746, -26.605685) (-35.763794, -26.605613) (-35.763844, -26.605521) (-35.76391, -26.605408) (-35.763995, -26.605258) (-35.764102, -26.605071) (-35.764272, -26.604771) (-35.764484, -26.604396) (-35.764735, -26.603944) (-35.764985, -26.603492) (-35.765314, -26.602889) (-35.765721, -26.602134) (-35.7662, -26.601224) (-35.766828, -26.600009) (-35.767591, -26.598484) (-35.768473, -26.596644) (-35.769322, -26.594794) (-35.770136, -26.592936) (-35.771176, -26.590451) (-35.772391, -26.587325) (-35.773718, -26.583541) (-35.774912, -26.579732) (-35.776324, -26.574635) (-35.777764, -26.568214) (-35.778974, -26.560446) (-35.779672, -26.552656) (-35.779864, -26.544867) (-35.779556, -26.537105) (-35.778491, -26.526834) (-35.775942, -26.514165) (-35.770989, -26.499467) (-35.764197, -26.485473) (-35.755608, -26.472381) (-35.741751, -26.456282) (-35.72888, -26.446343) (-35.719566, -26.440965) knots 0 0 0 0 0.00000162 0.00000648 0.00001296 0.00002591 0.00003886 0.00005181 0.00007769 0.00010357 0.00015528 0.00020695 0.00025856 0.00031013 0.00041314 0.00051596 0.0006186 0.00082338 0.00102748 0.00123095 0.00143381 0.00163608 0.00203896 0.00243981 0.00283881 0.00323614 0.00402628 0.00481152 0.00559287 0.00637121 0.00714727 0.00792172 0.00946727 0.01101283 0.01256256 0.01412145 0.01569602 0.01892257 0.01892257 0.01892257 0.01892257
  line L29 (-35.719566, -26.440965) -> (-33.763426, -25.311595)
  spline S65 degree 3 poles (-33.763426, -25.311595) (-33.763384, -25.311584) (-33.763315, -25.311525) (-33.763163, -25.311447) (-33.762902, -25.311292) (-33.762527, -25.311081) (-33.762076, -25.310827) (-33.761475, -25.310491) (-33.760721, -25.310077) (-33.759513, -25.309427) (-33.757996, -25.308635) (-33.756165, -25.307718) (-33.754324, -25.306836) (-33.751862, -25.305706) (-33.748762, -25.304378) (-33.745006, -25.302917) (-33.739972, -25.301151) (-33.733614, -25.299274) (-33.725895, -25.297543) (-33.718127, -25.296332) (-33.710336, -25.295634) (-33.699969, -25.295379) (-33.687051, -25.296305) (-33.671847, -25.299364) (-33.657146, -25.304319) (-33.638445, -25.313396) (-33.617143, -25.329422) (-33.604024, -25.346431) (-33.598646, -25.355745) knots 0 0 0 0 0.00001296 0.00002591 0.00005181 0.00010358 0.00015529 0.00020696 0.00031016 0.00041317 0.00061864 0.00082343 0.00102754 0.00123102 0.00163616 0.00203906 0.00243992 0.00323615 0.0040263 0.00481154 0.0055929 0.00637123 0.00792096 0.00946652 0.0110121 0.01256187 0.01568873 0.01891534 0.01891534 0.01891534 0.01891534
  line L30 (-33.598646, -25.355745) -> (-33.519276, -25.493225)
  spline S66 degree 3 poles (-33.519276, -25.493225) (-33.519265, -25.493267) (-33.519206, -25.493335) (-33.519128, -25.493488) (-33.518973, -25.493748) (-33.518762, -25.494124) (-33.518507, -25.494574) (-33.518172, -25.495176) (-33.517758, -25.495929) (-33.517108, -25.497138) (-33.516316, -25.498654) (-33.515399, -25.500486) (-33.514517, -25.502326) (-33.513387, -25.504789) (-33.512059, -25.507889) (-33.510598, -25.511645) (-33.508832, -25.516678) (-33.506955, -25.523037) (-33.505224, -25.530756) (-33.504013, -25.538524) (-33.503315, -25.546315) (-33.503059, -25.556682) (-33.503985, -25.569599) (-33.507045, -25.584804) (-33.512, -25.599505) (-33.521077, -25.618206) (-33.537103, -25.639508) (-33.554112, -25.652627) (-33.563426, -25.658005) knots 0 0 0 0 0.00001296 0.00002591 0.00005181 0.00010358 0.00015529 0.00020696 0.00031016 0.00041317 0.00061864 0.00082343 0.00102754 0.00123102 0.00163616 0.00203906 0.00243992 0.00323615 0.0040263 0.00481154 0.0055929 0.00637123 0.00792096 0.00946652 0.0110121 0.01256187 0.01568873 0.01891534 0.01891534 0.01891534 0.01891534
  line L31 (-33.563426, -25.658005) -> (-35.519566, -26.787375)
  spline S67 degree 3 poles (-35.519566, -26.787375) (-35.519607, -26.787386) (-35.519676, -26.787445) (-35.519829, -26.787523) (-35.520089, -26.787678) (-35.520465, -26.787889) (-35.520915, -26.788143) (-35.521517, -26.788479) (-35.52227, -26.788893) (-35.523478, -26.789543) (-35.524995, -26.790335) (-35.526826, -26.791252) (-35.528667, -26.792134) (-35.531129, -26.793264) (-35.534229, -26.794592) (-35.537986, -26.796053) (-35.543019, -26.797818) (-35.549377, -26.799696) (-35.557097, -26.801427) (-35.564864, -26.802638) (-35.572655, -26.803336) (-35.583022, -26.803591) (-35.595939, -26.802665) (-35.611143, -26.799606) (-35.625843, -26.794651) (-35.644543, -26.785574) (-35.665842, -26.769548) (-35.678959, -26.752539) (-35.684336, -26.743225) knots 0 0 0 0 0.00001296 0.00002591 0.00005181 0.00010358 0.00015529 0.00020696 0.00031016 0.00041317 0.00061864 0.00082343 0.00102754 0.00123102 0.00163616 0.00203906 0.00243992 0.00323614 0.00402629 0.00481153 0.00559287 0.0063712 0.00792089 0.0094664 0.01101191 0.01256159 0.01568823 0.01891458 0.01891458 0.01891458 0.01891458
  line L32 (-15.688936, -15.198875) -> (-15.768316, -15.061395)
  spline S68 degree 3 poles (-15.768316, -15.061395) (-15.768316, -15.061373) (-15.768353, -15.06134) (-15.768388, -15.061263) (-15.768468, -15.061134) (-15.768573, -15.060946) (-15.768702, -15.060721) (-15.768872, -15.060421) (-15.769084, -15.060046) (-15.769419, -15.059444) (-15.769833, -15.058691) (-15.770321, -15.057784) (-15.7708, -15.056874) (-15.771428, -15.055659) (-15.772191, -15.054134) (-15.773073, -15.052294) (-15.774203, -15.049831) (-15.775531, -15.046731) (-15.776991, -15.042975) (-15.778318, -15.039191) (-15.779512, -15.035382) (-15.780924, -15.030285) (-15.782364, -15.023864) (-15.783574, -15.016096) (-15.784272, -15.008305) (-15.784527, -14.997938) (-15.783602, -14.985021) (-15.780542, -14.969816) (-15.775589, -14.955116) (-15.766513, -14.936414) (-15.750488, -14.915112) (-15.73348, -14.901993) (-15.724166, -14.896615) knots 0 0 0 0 0.00000648 0.00001296 0.00002591 0.00005181 0.00007769 0.00010357 0.00015528 0.00020695 0.00031013 0.00041314 0.00051596 0.0006186 0.00082337 0.00102748 0.00123095 0.00163607 0.00203895 0.0024398 0.0028388 0.00323612 0.00402626 0.00481151 0.00559286 0.00637119 0.00792092 0.00946647 0.01101202 0.01256176 0.01568853 0.01891509 0.01891509 0.01891509 0.01891509
  line L33 (-15.724166, -14.896615) -> (-13.768026, -13.767245)
  spline S69 degree 3 poles (-13.768026, -13.767245) (-13.767984, -13.767234) (-13.767915, -13.767175) (-13.767763, -13.767097) (-13.767502, -13.766942) (-13.767127, -13.766731) (-13.766676, -13.766477) (-13.766075, -13.766141) (-13.765321, -13.765727) (-13.764113, -13.765077) (-13.762596, -13.764285) (-13.760765, -13.763368) (-13.758924, -13.762486) (-13.756462, -13.761356) (-13.753362, -13.760028) (-13.749606, -13.758567) (-13.744572, -13.756801) (-13.738214, -13.754924) (-13.730495, -13.753193) (-13.722727, -13.751982) (-13.714936, -13.751284) (-13.704569, -13.751029) (-13.691651, -13.751955) (-13.676447, -13.755014) (-13.661746, -13.759969) (-13.643045, -13.769046) (-13.621743, -13.785072) (-13.608624, -13.802081) (-13.603246, -13.811395) knots 0 0 0 0 0.00001296 0.00002591 0.00005181 0.00010358 0.00015529 0.00020696 0.00031016 0.00041317 0.00061864 0.00082343 0.00102754 0.00123102 0.00163616 0.00203906 0.00243992 0.00323615 0.0040263 0.00481154 0.0055929 0.00637123 0.00792096 0.00946652 0.0110121 0.01256187 0.01568873 0.01891534 0.01891534 0.01891534 0.01891534
  line L34 (-13.603246, -13.811395) -> (-13.523876, -13.948875)
  spline S70 degree 3 poles (-13.523876, -13.948875) (-13.523865, -13.948917) (-13.523806, -13.948985) (-13.523728, -13.949138) (-13.523573, -13.949398) (-13.523362, -13.949774) (-13.523107, -13.950224) (-13.522772, -13.950826) (-13.522358, -13.951579) (-13.521708, -13.952788) (-13.520916, -13.954304) (-13.519999, -13.956136) (-13.519117, -13.957976) (-13.517987, -13.960439) (-13.516659, -13.963539) (-13.515198, -13.967295) (-13.513432, -13.972328) (-13.511555, -13.978687) (-13.509824, -13.986406) (-13.508613, -13.994174) (-13.507915, -14.001965) (-13.507659, -14.012332) (-13.508585, -14.025249) (-13.511645, -14.040454) (-13.5166, -14.055155) (-13.525677, -14.073856) (-13.541703, -14.095158) (-13.558712, -14.108277) (-13.568026, -14.113655) knots 0 0 0 0 0.00001296 0.00002591 0.00005181 0.00010358 0.00015529 0.00020696 0.00031016 0.00041317 0.00061864 0.00082343 0.00102754 0.00123102 0.00163616 0.00203906 0.00243992 0.00323615 0.0040263 0.00481154 0.0055929 0.00637123 0.00792096 0.00946652 0.0110121 0.01256187 0.01568873 0.01891534 0.01891534 0.01891534 0.01891534
  line L35 (-13.568026, -14.113655) -> (-15.524166, -15.243025)
  spline S71 degree 3 poles (-15.524166, -15.243025) (-15.524207, -15.243036) (-15.524276, -15.243095) (-15.524429, -15.243173) (-15.524689, -15.243328) (-15.525065, -15.243539) (-15.525515, -15.243793) (-15.526117, -15.244129) (-15.52687, -15.244543) (-15.528078, -15.245193) (-15.529595, -15.245985) (-15.531426, -15.246902) (-15.533267, -15.247784) (-15.535729, -15.248914) (-15.538829, -15.250242) (-15.542586, -15.251703) (-15.547619, -15.253468) (-15.553977, -15.255346) (-15.561697, -15.257077) (-15.569464, -15.258288) (-15.577255, -15.258986) (-15.587622, -15.259241) (-15.600539, -15.258315) (-15.615743, -15.255256) (-15.630443, -15.250301) (-15.649143, -15.241224) (-15.670442, -15.225198) (-15.683559, -15.208189) (-15.688936, -15.198875) knots 0 0 0 0 0.00001296 0.00002591 0.00005181 0.00010358 0.00015529 0.00020696 0.00031016 0.00041317 0.00061864 0.00082343 0.00102754 0.00123102 0.00163616 0.00203906 0.00243992 0.00323614 0.00402629 0.00481153 0.00559287 0.0063712 0.00792089 0.0094664 0.01101191 0.01256159 0.01568823 0.01891458 0.01891458 0.01891458 0.01891458
  line L36 (-35.763716, -13.948865) -> (-35.684336, -13.811385)